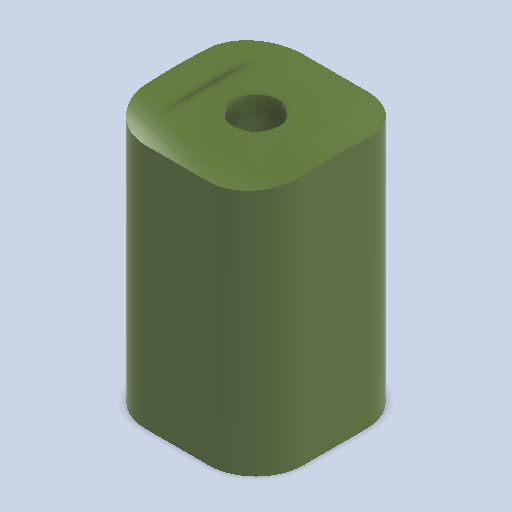
# Autodesk Inventor part: brush_holder_batt
Saved by Autodesk Inventor 2025 (Build 290162000, 162)
## iProperties
Created: 2026-08-13
Part Number: brush_holder_batt
Material: Ogólny
Document SubType Name: Modeling
Designer: zzapa
Density: 1 g/cm^3
Appearance: Ciemnooliwkowa
Author: zzapa
Autodesk Inventor part; units mm, degrees
ref_plane "YZ Plane" through (0, 0, 0) normal (1, 0, 0) x (0, 1, 0)
ref_plane "XZ Plane" through (0, 0, 0) normal (0, 1, 0) x (-1, 0, 0)
sketch "Szkic1" plane through (0, 0, 0) normal (1, 0, 0) x (0, 1, 0)
  line L0 (16, 5) -> (0, 5)
  line L1 (0, 5) -> (0, -5)
  line L2 (0, -5) -> (16, -5)
  line L3 (16, -5) -> (16, 5)
  line L4 (0, -7) -> (0, 7) projected
  point P0 (0, 0)
  dimension "d0" = 10
  dimension "d1" = 16
  constraints: 8 end point, 2 parallel, 1 horizontal, 1 midpoint, 1 perpendicular
  measures "d0" distance of L2.end L0.start
  measures "d1" distance of L1.end L2.end
extrude "Wyciągnięcie proste1" add sketch "Szkic1" along normal blind 10
sketch "Szkic2" plane through (10, 0, 0) normal (1, 0, 0) x (0, 0, -1)
  circle A0 centre (0, -14.15) radius 30.15
  line L0 (5, 16) -> (-5, 16) projected
  line L1 (0, -60.8) -> (0, 28.8) projected
  point P0 (0, 0)
  dimension "d4" = 60.3
  constraints: 1 centre point, 1 point on line, 1 tangent
  measures "d4" diameter of A0
extrude "Wyciągnięcie proste2" cut sketch "Szkic2" against normal through all keep common part
ref_plane "Płaszczyzna konstrukcyjna2" through (5, 0, 0) normal (-1, 0, 0) x (0, 0, 1)
sketch "Szkic3" plane through (5, 0, 0) normal (-1, 0, 0) x (0, 0, 1)
  arc A0 (5, 15.582516) -> (-5, 15.582516) centre (0, -14.15) ccw
  line L0 (0, -20.18) -> (0, 22.03)
  line L1 (-3, 16) -> (3, 16)
  line L2 (3, 16) -> (3, 15.850375)
  line L3 (3, 15.850375) -> (-3, 15.850375)
  line L4 (-3, 15.850375) -> (-3, 16)
  point P0 (0, 0)
  point P1 (0, 16)
  dimension "d7" = 6
  constraints: 8 end point, 2 parallel, 1 horizontal, 1 midpoint, 1 perpendicular, 1 point on circle, 1 point on line, 1 tangent
  measures "d7" distance of L1.start L1.end
sketch "Szkic3 outline for Wyciągnięcie proste3" plane through (5, 0, 0) normal (-1, 0, 0) x (0, 0, 1)
  line L0 (-3, 16) -> (-3, 15.850375)
  line L1 (3, 16) -> (-3, 16)
  line L2 (3, 15.850375) -> (3, 16)
  line L3 (-3, 15.850375) -> (3, 15.850375)
extrude "Wyciągnięcie proste3" cut sketch "Szkic3 outline for Wyciągnięcie proste3" along normal mid plane 6
sketch "Szkic4" plane through (2, 15.850375, 3) normal (0, 1, 0) x (1, 0, 0)
  line L0 (0, 6) -> (6, 6) projected
  line L1 (6, 0) -> (0, 0) projected
  line L2 (3, 6) -> (3, 0)
  point P0 (-2, 3)
  point P1 (3, 3)
  point P2 (3, 3)
  constraints: 3 midpoint, 2 end point, 1 coincident, 1 vertical
hole "Otwór1" at (5, 15.850375, 0) direction (0, -1, 0) diameter 2.9 depth 5
sketch "Szkic5" plane through (0, 0, -5) normal (0, -1, 0) x (1, 0, 0)
  line L0 (0, 10) -> (10, 10) projected
  line L1 (5, 10) -> (5, 0)
  line L2 (0, 0) -> (10, 0) projected
  point P0 (0, 5)
  point P1 (5, 5)
  constraints: 3 midpoint, 2 end point
hole "Otwór2" at (5, 0, 0) direction (0, 1, 0) diameter 4.5 depth 10
sketch "Szkic6" plane through (0, 0, 0) normal (-1, 0, 0) x (0, 0, 1)
  line L0 (-0.78917, 10) -> (0.78917, 10)
  line L1 (0.78917, 10) -> (0.78917, 0)
  line L2 (0.78917, 0) -> (-0.78917, 0)
  line L3 (-0.78917, 0) -> (-0.78917, 10)
  line L4 (5, 0) -> (-5, 0)
  line L5 (-2.25, 10) -> (2.25, 10)
  point P0 (0, 0)
  point P1 (0, 0)
  point P2 (2, 0)
  point P3 (-2, 0)
  constraints: 8 end point, 2 midpoint, 2 parallel, 1 collinear, 1 horizontal, 1 perpendicular
extrude "Wyciągnięcie proste4" cut sketch "Szkic6" against normal up to surface
fillet "Zaokrąglenie2" radius 3 4 edges at (0, 7.7913, -5) (0, 7.7913, 5) (10, 7.7913, 5) (10, 7.7913, -5)
fillet "Zaokrąglenie3" radius 0.5 4 edges at (0, 5, -0.7892) (0, 5, 0.7892) (2.8929, 5, -0.7892) (2.8929, 5, 0.7892)
equation "\"d0\" = brush_holder_batt_length"
equation "\"d1\" = brush_holder_batt_width"
equation "\"d2\" = brush_holder_batt_depth"
equation "\"d4\" = 2 * brush_holder_batt_arc_r"
equation "\"d7\" = brush_holder_batt_insert_flat_length"
equation "\"d8\" = brush_holder_batt_insert_flat_depth"
equation "\"d10\" = insert_m2_d"
equation "\"d12\" = insert_m2_pocket_D"
equation "\"d13\" = insert_m2_pocket_nut_h"
equation "\"d17\" = brush_holder_batt_brush_hole_d"
equation "\"d22\" = brush_holder_batt_brush_hole_h"
equation "\"insert_m2_d\" = 2.9"
equation "\"insert_m2_h\" = 7"
equation "\"insert_m2_corner\" = 0.5"
equation "\"insert_m2_pocket_d\" = 2.6"
equation "\"insert_m2_pocket_D\" = 4.5"
equation "\"insert_m2_pocket_nut_h\" = 1.5"
equation "\"stator_r_out\" = 30.15"
equation "\"stator_out_d\" = 3.2"
equation "\"stator_h\" = 45"
equation "\"stator_radial_screw_d\" = 4"
equation "\"stator_radial_screw_pos\" = 4"
equation "\"mag_size_x\" = 7"
equation "\"mag_size_y\" = 3"
equation "\"mag_corner_r\" = 0.4"
equation "\"magnet_ring_r\" = 26.95"
equation "\"magnet_ring_d\" = 3.3"
equation "\"magnet_ring_h\" = 36"
equation "\"magnet_ring_pocket_mag_size_x\" = 7.1"
equation "\"magnet_ring_pocket_mag_size_y\" = 3.1"
equation "\"magnet_ring_pocket_mag_size_z\" = 10.1"
equation "\"magnet_ring_pocket_radial_cut\" = 1.4"
equation "\"magnet_ring_insert_part_lengthen\" = 8"
equation "\"magnet_ring_insert_part_axial_flat_cut\" = 0.17"
equation "\"magnet_ring_insert_pos\" = 4"
equation "\"casing_d\" = 3"
equation "\"casing_r_in\" = 30.15"
equation "\"casing_lock_hole_r\" = 14.25"
equation "\"casing_lock_h\" = 8"
equation "\"casing_stator_fix_r\" = 23"
equation "\"casing_stator_fix_h\" = 6"
equation "\"casing_sidebar_length\" = 3"
equation "\"casing_vent_hole_length\" = 4"
equation "\"casing_vent_hole_width\" = 6"
equation "\"casing_head_insert_r\" = 19"
equation "\"casing_radial_stator_insert_pos\" = 18.1"
equation "\"casing_cart_hole_ang\" = 90deg"
equation "\"casing_cart_hole_width\" = 2.6"
equation "\"casing_cart_hole_corner\" = 1"
equation "\"rotor_out_r\" = 22.5"
equation "\"rotor_coil_groove_in_r\" = 17"
equation "\"rotor_coil_groove_ang\" = 18deg"
equation "\"rotor_core_r\" = 14.97"
equation "\"rotor_coil_groove_in_correction_r\" = 18"
equation "\"rotor_plastic_h\" = 32"
equation "\"rotor_teeth_d\" = 1.5"
equation "\"rotor_plastic_insert_r\" = 37"
equation "\"shaft_d\" = 8"
equation "\"shaft_lock_1_d\" = 8.1"
equation "\"shaft_lock_1_D\" = 44"
equation "\"shaft_lock_1_h1\" = 3.5"
equation "\"shaft_lock_1_corner\" = 2"
equation "\"shaft_lock_1_rotor_insert_grove_d_in\" = 36"
equation "\"shaft_lock_1_rotor_insert_grove_width_out\" = 5.5"
equation "\"shaft_lock_1_rotor_insert_grove_width_in\" = 7.6"
equation "\"shaft_lock_1_rotor_insert_r\" = 37"
equation "\"shaft_lock_1_shaft_insert_axial_cut_out_width\" = 12"
equation "\"shaft_lock_1_shaft_insert_axial_cut_in_width\" = 5.4"
equation "\"shaft_lock_1_shaft_insert_pos\" = 2.5"
equation "\"shaft_lock_1_shaft_insert_corner\" = 2"
equation "\"shaft_lock_1_shaft_insert_corner_finish\" = 0.5"
equation "\"shaft_lock_2_d\" = 8.1"
equation "\"shaft_lock_2_D\" = 44"
equation "\"shaft_lock_2_h1\" = 3.5"
equation "\"shaft_lock_2_corner\" = 2"
equation "\"shaft_lock_2_rotor_insert_grove_d_in\" = 36"
equation "\"shaft_lock_2_rotor_insert_grove_width_out\" = 5.5"
equation "\"shaft_lock_2_rotor_insert_grove_width_in\" = 7.6"
equation "\"shaft_lock_2_rotor_insert_r\" = 37"
equation "\"shaft_lock_2_shaft_insert_axial_cut_out_width\" = 12"
equation "\"shaft_lock_2_shaft_insert_axial_cut_in_width\" = 5.4"
equation "\"shaft_lock_2_shaft_insert_pos\" = 2.5"
equation "\"shaft_lock_2_shaft_insert_corner\" = 2"
equation "\"shaft_lock_2_shaft_insert_corner_finish\" = 0.5"
equation "\"commutator_plastic_shaft_d\" = 8.1"
equation "\"commutator_plastic_h\" = 17"
equation "\"commutator_plastic_insert_cut_deepness\" = 0.5"
equation "\"commutator_plastic_insert_cut_length\" = 6"
equation "\"commutator_plastic_insert_pos\" = 3"
equation "\"commutator_plate_D\" = 22"
equation "\"commutator_plate_d\" = 1"
equation "\"commutator_plate_ang\" = 55deg"
equation "\"commutator_plate_h\" = 17"
equation "\"commutator_plate_insert_pos\" = 3"
equation "\"sleeve_in_r\" = 11.1"
equation "\"sleeve_d\" = 3"
equation "\"sleeve_h\" = 7"
equation "\"sleeve_cup_r\" = 22"
equation "\"sleeve_cup_h\" = 4.5"
equation "\"sleeve_head_insert_r\" = 19"
equation "\"rotor_sleeve_in_D\" = 8.15"
equation "\"rotor_sleeve_out_D\" = 10.5"
equation "\"rotor_sleeve_h\" = 32"
equation "\"carbon_brush_batt_d\" = 4"
equation "\"carbon_brush_batt_h\" = 8"
equation "\"brush_cart_outer_holder_width\" = 5.5"
equation "\"brush_cart_outer_holder_arc_r\" = 33.15"
equation "\"brush_cart_outer_holder_arc_pos\" = 1.5"
equation "\"brush_holder_batt_length\" = 10"
equation "\"brush_holder_batt_width\" = 16"
equation "\"brush_holder_batt_depth\" = 10"
equation "\"brush_holder_batt_arc_r\" = 30.15"
equation "\"brush_holder_batt_insert_flat_length\" = 6"
equation "\"brush_holder_batt_insert_flat_depth\" = 6"
equation "\"brush_holder_batt_insert_flat_width\" = 2"
equation "\"brush_holder_batt_brush_hole_d\" = 4.5"
equation "\"brush_holder_batt_brush_hole_h\" = 10"
equation "\"casing_backsleeve_insert_pos\" = 4.9"
equation "\"casing_cart_hole_pos\" = 17"
equation "\"casing_sleeve_cut_d\" = 46"
equation "\"casing_sleeve_cut_h\" = 4"
equation "\"name_plate_D\" = 45"
equation "\"name_plate_d\" = 28"
equation "\"name_plate_insert_r\" = 19"
equation "\"sleeve_bearing_material_lock_h\" = 2"
equation "\"back_sleeve_D\" = 66"
equation "\"back_sleeve_d\" = 22.2"
equation "\"back_sleeve_h\" = 5"
equation "\"commutator_back_plate_lock_h\" = 2"
equation "\"commutator_back_plate_lock_r\" = 23"
equation "\"commutator_plastic_back_plate_lock_r\" = 11.9"
